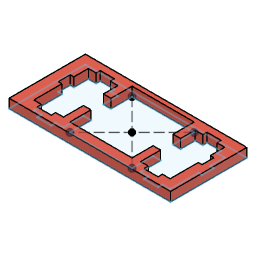
Adalyn (Autodesk Fusion 360 archive; units mm, degrees)
design "Component8"
Autodesk Fusion 360 part; units mm, degrees
sketch "sketch 356" plane through (0, 1.5, 0) normal (0, 1, 0) x (-1, 0, 0)
  line L0 (-100.825, -30.4246) -> (-100.825, -31.4057)
  line L1 (-100.825, -31.4057) -> (-99.1, -31.4057)
  line L2 (-99.1, -31.4057) -> (-99.1, -37.6756)
  line L3 (-99.1, -37.6756) -> (-98.274, -37.6756)
  line L4 (-98.274, -37.6756) -> (-98.274, -40.3257)
  line L5 (-98.274, -40.3257) -> (-99.1, -40.3257)
  line L6 (-99.1, -40.3257) -> (-99.1, -43.5557)
  line L7 (-99.1, -43.5557) -> (-100.825, -43.5557)
  line L8 (-100.825, -43.5557) -> (-100.825, -44.475)
  line L9 (-100.825, -44.475) -> (-103.974, -44.475)
  line L10 (-103.974, -44.475) -> (-103.974, -43.5557)
  line L11 (-103.974, -43.5557) -> (-105.699, -43.5557)
  line L12 (-105.699, -43.5557) -> (-105.699, -40.3257)
  line L13 (-105.699, -40.3257) -> (-107.375, -40.3257)
  line L14 (-107.375, -40.3257) -> (-107.375, -45.0247)
  line L15 (-107.375, -45.0247) -> (-121.224, -45.0247)
  line L16 (-121.224, -45.0247) -> (-121.224, -40.3257)
  line L17 (-121.224, -40.3257) -> (-122.9, -40.3257)
  line L18 (-122.9, -40.3257) -> (-122.9, -43.5557)
  line L19 (-122.9, -43.5557) -> (-124.625, -43.5557)
  line L20 (-124.625, -43.5557) -> (-124.625, -44.475)
  line L21 (-124.625, -44.475) -> (-127.774, -44.475)
  line L22 (-127.774, -44.475) -> (-127.774, -43.5557)
  line L23 (-127.774, -43.5557) -> (-129.499, -43.5557)
  line L24 (-129.499, -43.5557) -> (-129.499, -40.3257)
  line L25 (-129.499, -40.3257) -> (-130.325, -40.3257)
  line L26 (-130.325, -40.3257) -> (-130.325, -37.6756)
  line L27 (-130.325, -37.6756) -> (-129.499, -37.6756)
  line L28 (-129.499, -37.6756) -> (-129.499, -31.4057)
  line L29 (-129.499, -31.4057) -> (-127.774, -31.4057)
  line L30 (-127.774, -31.4057) -> (-127.774, -30.4246)
  line L31 (-127.774, -30.4246) -> (-124.625, -30.4246)
  line L32 (-124.625, -30.4246) -> (-124.625, -31.4057)
  line L33 (-124.625, -31.4057) -> (-122.9, -31.4057)
  line L34 (-122.9, -31.4057) -> (-122.9, -35.8747)
  line L35 (-122.9, -35.8747) -> (-121.224, -35.8747)
  line L36 (-121.224, -35.8747) -> (-121.224, -31.1757)
  line L37 (-121.224, -31.1757) -> (-107.375, -31.1757)
  line L38 (-107.375, -31.1757) -> (-107.375, -35.8747)
  line L39 (-107.375, -35.8747) -> (-105.699, -35.8747)
  line L40 (-105.699, -35.8747) -> (-105.699, -31.4057)
  line L41 (-105.699, -31.4057) -> (-103.974, -31.4057)
  line L42 (-103.974, -31.4057) -> (-103.974, -30.4246)
  line L43 (-103.974, -30.4246) -> (-100.825, -30.4246)
  line L44 (-132, -29) -> (-96, -29)
  line L45 (-132, -46) -> (-132, -29)
  line L46 (-96, -46) -> (-132, -46)
  line L47 (-96, -29) -> (-96, -46)
extrude "Extrude1" add sketch "sketch 356" along normal blind 2
sketch "Sketch1" plane through (0, 1.5, 0) normal (0, 1, 0) x (-1, 0, 0)
  line L0 (-121.224, -45.0247) -> (-107.375, -31.1757) construction
  line L1 (-107.375, -45.0247) -> (-121.224, -31.1757) construction
  point P0 (-121.224, -45.0247)
  point P1 (-107.375, -45.0247)
  point P2 (-107.375, -31.1757)
  point P3 (-121.224, -31.1757)
  point P4 (-114.2995, -38.1002)
  constraint coincident P0 L0.start
  constraint coincident P2 L0.end
  constraint coincident P1 L1.start
  constraint coincident P3 L1.end
  constraint midpoint L0 P4
